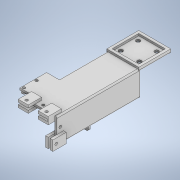
# Autodesk Inventor part: carriageEndL
Saved by Autodesk Inventor 2020 (Build 240168000, 168)
## iProperties
Created: 2020-01-10
Part Number: carriageEndL
Material: Generic
Document SubType Name: Modeling
Designer: PAB
Density: 1 g/cm^3
Appearance: Default
Author: PAB
Autodesk Inventor part; units mm, degrees
ref_plane "YZ Plane" through (0, 0, 0) normal (1, 0, 0) x (0, 1, 0)
ref_plane "XZ Plane" through (0, 0, 0) normal (0, 1, 0) x (-1, 0, 0)
ref_plane "XY Plane" through (0, 0, 0) normal (0, 0, 1) x (1, 0, 0)
sketch "Sketch1" plane through (0, 0, 0) normal (0, 1, 0) x (-1, 0, 0)
  line L0 (24, 138) -> (-24, 138)
  line L1 (-24, 138) -> (-24, -138)
  line L2 (-24, -138) -> (24, -138)
  line L3 (24, -138) -> (24, 138)
  point P0 (0, 0)
  dimension "d0" = 48
  dimension "d1" = 276
  constraints: 8 end point, 2 parallel, 1 horizontal, 1 perpendicular
  measures "d0" distance of L2.end L1.end
  measures "d1" distance of L1.end L0.end
extrude "Extrusion1" add sketch "Sketch1" along normal blind 3
sketch "Sketch2" plane through (0, 3, 0) normal (0, 1, 0) x (1, 0, 0)
  line L0 (-24, 138) -> (-24, -138) projected
  line L1 (-24, -138) -> (-20, -138)
  line L2 (-20, -138) -> (-20, -90)
  line L3 (-20, -90) -> (-24, -90)
  line L4 (-24, -90) -> (-24, -138)
  line L5 (24, -138) -> (24, 138) projected
  line L6 (-20, -90) -> (24, -90)
  line L7 (24, -90) -> (24, -94)
  line L8 (24, -94) -> (-20, -94)
  line L9 (-20, -94) -> (-20, -90)
  line L10 (-24, -138) -> (24, -138) projected
  line L11 (24, -94) -> (20, -94)
  line L12 (20, -94) -> (20, -138)
  line L13 (20, -138) -> (24, -138)
  line L14 (24, -138) -> (24, -94)
  line L15 (20, -138) -> (-20, -138)
  line L16 (-20, -138) -> (-20, -134)
  line L17 (-20, -134) -> (20, -134)
  line L18 (20, -134) -> (20, -138)
  point P0 (0, 0)
  point P1 (20, -134)
  dimension "d4" = 4
  dimension "d5" = 48
  dimension "d6" = 4
  dimension "d7" = 4
  dimension "d8" = 4
  constraints: 32 end point, 8 parallel, 4 horizontal, 4 perpendicular, 3 point on line
  measures "d4" distance of L3.end L2.end
  measures "d5" distance of L2.end L1.end
  measures "d6" distance of L6.end L7.end
  measures "d7" distance of L13.end L12.end
  measures "d8" distance of L15.end L16.end
extrude "Extrusion2" add sketch "Sketch2" along normal blind 3 contours L3 L2 L1 L0 | L6 L5 L8 L2 | L2 L17 L12 L10 | L12 L8 L5 L10
mirror "Mirror1" about plane through (0, 0, 0) normal (0, 0, 1) of "Extrusion2"
sketch "Sketch3" plane through (0, 0, 0) normal (0, -1, 0) x (1, 0, 0)
  line L0 (24, -90) -> (-24, -90) projected
  line L1 (24, 138) -> (24, -138) projected
  line L2 (-24, -90) -> (24, -90)
  line L3 (24, -90) -> (24, -93)
  line L4 (24, -93) -> (-24, -93)
  line L5 (-24, -93) -> (-24, -90)
  line L6 (-24, 90) -> (24, 90) projected
  line L7 (24, 90) -> (21, 90)
  line L8 (21, 90) -> (21, -90)
  line L9 (21, -90) -> (24, -90)
  line L10 (24, -90) -> (24, 90)
  line L11 (-24, 90) -> (24, 90)
  line L12 (24, 90) -> (24, 93)
  line L13 (24, 93) -> (-24, 93)
  line L14 (-24, 93) -> (-24, 90)
  point P0 (0, 0)
  dimension "d11" = 3
  dimension "d12" = 3
  dimension "d13" = 3
  constraints: 24 end point, 6 parallel, 3 horizontal, 3 perpendicular, 3 point on line
  measures "d11" distance of L2.end L3.end
  measures "d12" distance of L9.end L8.end
  measures "d13" distance of L12.end L11.end
extrude "Extrusion3" add sketch "Sketch3" along normal blind 35
sketch "Sketch4" plane through (-24, 0, -90) normal (0, 0, 1) x (1, 0, 0)
  line L0 (0, -35) -> (45, -35) projected
  line L1 (45, 0) -> (45, -35) projected
  line L2 (0, -35) -> (45, -35)
  line L3 (45, -35) -> (45, -31)
  line L4 (45, -31) -> (0, -31)
  line L5 (0, -31) -> (0, -35)
  point P0 (24, 0)
  dimension "d16" = 4
  constraints: 8 end point, 2 parallel, 1 horizontal, 1 perpendicular, 1 point on line
  measures "d16" distance of L3.end L2.end
extrude "Extrusion4" add sketch "Sketch4" along normal blind 8
sketch "Sketch5" plane through (-24, -31, -90) normal (0, 1, 0) x (1, 0, 0)
  line L0 (0, -8) -> (45, -8) projected
  line L1 (45, 0) -> (45, -8) projected
  line L2 (0, -8) -> (45, -8)
  line L3 (45, -8) -> (45, -4)
  line L4 (45, -4) -> (0, -4)
  line L5 (0, -4) -> (0, -8)
  point P0 (24, -90)
  dimension "d19" = 4
  constraints: 8 end point, 2 parallel, 1 horizontal, 1 midpoint, 1 perpendicular
  measures "d19" distance of L3.end L2.end
extrude "Extrusion5" add sketch "Sketch5" along normal blind 4
sketch "Sketch6" plane through (0, 0, 0) normal (0, -1, 0) x (1, 0, 0)
  line L0 (21, -86) -> (-24, -86) projected
  line L1 (-24, -82) -> (21, -82)
  line L2 (21, -82) -> (21, -86)
  line L3 (21, -86) -> (-24, -86)
  line L4 (-24, -86) -> (-24, -82)
  point P0 (0, 0)
  dimension "d22" = 4
  constraints: 8 end point, 2 parallel, 1 horizontal, 1 perpendicular
  measures "d22" distance of L1.end L0.start
extrude "Extrusion6" add sketch "Sketch6" along normal blind 4
mirror "Mirror2" about plane through (0, 0, 0) normal (0, 0, 1) of "Extrusion6", "Extrusion5", "Extrusion4"
sketch "Sketch7" plane through (0, 0, 0) normal (0, -1, 0) x (1, 0, 0)
  circle A0 centre (-14, -127) radius 3
  circle A1 centre (14, -127) radius 3
  circle A2 centre (14, -101) radius 3
  circle A3 centre (-14, -101) radius 3
  line L0 (-20, -94) -> (20, -94) projected
  line L1 (20, -94) -> (20, -134) projected
  line L2 (-20, -134) -> (-20, -94) projected
  point P0 (0, 0)
  dimension "d25" = 6
  dimension "d26" = 6
  dimension "d27" = 6
  dimension "d28" = 6
  dimension "d135" = 28
  dimension "d136" = 26
  dimension "d137" = 28
  dimension "d138" = 26
  dimension "d139" = 7
  dimension "d140" = 7
  dimension "d141" = 6
  dimension "d142" = 6
  constraints: 4 centre point
  measures "d25" diameter of A0
  measures "d26" diameter of A1
  measures "d27" diameter of A2
  measures "d28" diameter of A3
  measures "d135" distance of A2.centre A3.centre
  measures "d136" distance of A1.centre A2.centre
  measures "d137" distance of A1.centre A0.centre
  measures "d138" distance of A3.centre A0.centre
  measures "d139" distance from line of L0 A3.centre
  measures "d140" distance from line of L0 A2.centre
  measures "d141" distance from line of L1 A2.centre
  measures "d142" distance from line of L2 A0.centre
extrude "Extrusion7" cut sketch "Sketch7" against normal blind 4
mirror "Mirror3" about plane through (0, 0, 0) normal (0, 0, 1) of "Extrusion7"
sketch "Sketch8" plane through (0, 0, 0) normal (0, -1, 0) x (1, 0, 0)
  line L0 (21, 82) -> (21, -82) projected
  line L1 (-24, -82) -> (-24, 82) projected
  line L2 (21, -20) -> (-24, -20)
  line L3 (-24, -20) -> (-24, -17)
  line L4 (-24, -17) -> (21, -17)
  line L5 (21, -17) -> (21, -20)
  point P0 (0, 0)
  dimension "d31" = 3
  constraints: 8 end point, 2 parallel, 2 point on line, 1 horizontal, 1 perpendicular
  measures "d31" distance of L2.end L3.end
extrude "Extrusion8" add sketch "Sketch8" along normal blind 42.3
sketch "Sketch9" plane through (21, 0, -20) normal (0, 0, -1) x (-1, 0, 0)
  circle A0 centre (39.35, -5.65) radius 4
  circle A1 centre (39.35, -36.65) radius 4
  circle A2 centre (8.35, -5.65) radius 4
  circle A3 centre (8.35, -36.65) radius 4
  point P0 (21, 0)
  dimension "d34" = 8
  dimension "d35" = 8
  dimension "d36" = 8
  dimension "d37" = 8
  constraints: 4 centre point
  measures "d34" diameter of A0
  measures "d35" diameter of A1
  measures "d36" diameter of A2
  measures "d37" diameter of A3
extrude "Extrusion9" add sketch "Sketch9" along normal blind 3
sketch "Sketch10" plane through (-18.35, -36.65, -23) normal (0, 0, -1) x (-1, 0, 0)
  circle A0 centre (0, 0) radius 3
  circle A1 centre (0, 31) radius 4 projected
  circle A2 centre (0, 31) radius 3
  circle A3 centre (-31, 0) radius 4 projected
  circle A4 centre (-31, 0) radius 3
  circle A5 centre (-31, 31) radius 4 projected
  circle A6 centre (-31, 31) radius 3
  point P0 (-18.35, 36.65)
  dimension "d40" = 6
  dimension "d41" = 6
  dimension "d42" = 6
  dimension "d43" = 6
  constraints: 4 centre point, 3 coincident
  measures "d40" diameter of A0
  measures "d41" diameter of A2
  measures "d42" diameter of A4
  measures "d43" diameter of A6
extrude "Extrusion10" cut sketch "Sketch10" against normal blind 2 contours A0 | A2 | A4 | A6
sketch "Sketch11" plane through (21, 0, -20) normal (0, 0, -1) x (-1, 0, 0)
  circle A0 centre (23.85, -21.15) radius 12.5
  circle A1 centre (39.35, -36.65) radius 3 projected
  circle A2 centre (39.35, -36.65) radius 2
  circle A3 centre (8.35, -36.65) radius 3 projected
  circle A4 centre (8.35, -36.65) radius 2
  circle A5 centre (8.35, -5.65) radius 4 projected
  circle A6 centre (8.35, -5.65) radius 2
  circle A7 centre (39.35, -5.65) radius 4 projected
  circle A8 centre (39.35, -5.65) radius 2
  point P0 (21, 0)
  dimension "d46" = 25
  dimension "d47" = 4
  dimension "d48" = 4
  dimension "d49" = 4
  dimension "d50" = 4
  constraints: 5 centre point, 4 coincident
  measures "d46" diameter of A0
  measures "d47" diameter of A2
  measures "d48" diameter of A4
  measures "d49" diameter of A6
  measures "d50" diameter of A8
extrude "Extrusion11" cut sketch "Sketch11" along normal mid plane 10 contours A0 | A2 | A4 | A6 | A8
sketch "Sketch20" plane through (0, 0, 0) normal (0, -1, 0) x (1, 0, 0)
  line L0 (-24, -90) -> (-24, 90) projected
  line L1 (-24, 138) -> (24, 138) projected
  line L2 (-24, 33) -> (24, 33)
  line L3 (24, 33) -> (24, 138)
  line L4 (24, 138) -> (-24, 138)
  line L5 (-24, 138) -> (-24, 33)
  point P0 (0, 0)
  constraints: 8 end point, 2 parallel, 1 horizontal, 1 perpendicular, 1 point on line
extrude "Extrusion20" cut sketch "Sketch20" along normal mid plane 100
sketch "Sketch21" plane through (0, 0, 0) normal (0, -1, 0) x (1, 0, 0)
  line L0 (-24, 23) -> (-9, 23)
  line L1 (-9, 23) -> (-9, 43)
  line L2 (-9, 43) -> (-24, 43)
  line L3 (-24, 43) -> (-24, 23)
  line L4 (6, 23) -> (21, 23)
  line L5 (21, 23) -> (21, 43)
  line L6 (21, 43) -> (6, 43)
  line L7 (6, 43) -> (6, 23)
  point P0 (0, 0)
  dimension "d86" = 15
  dimension "d87" = 20
  dimension "d88" = 15
  dimension "d89" = 20
  constraints: 16 end point, 4 parallel, 2 horizontal, 2 perpendicular
  measures "d86" distance of L2.end L1.end
  measures "d87" distance of L1.end L0.end
  measures "d88" distance of L6.end L5.end
  measures "d89" distance of L5.end L4.end
extrude "Extrusion21" add sketch "Sketch21" along normal blind 4 and the other way blind 7
sketch "Sketch24" plane through (0, -4, 0) normal (0, -1, 0) x (1, 0, 0)
  circle A0 centre (-16.5, 38) radius 2
  circle A1 centre (13.5, 38) radius 2
  circle A2 centre (-1.5, 28) radius 2
  point P0 (0, 0)
  dimension "d102" = 4
  dimension "d103" = 4
  dimension "d104" = 4
  constraints: 3 centre point
  measures "d102" diameter of A0
  measures "d103" diameter of A1
  measures "d104" diameter of A2
extrude "Extrusion24" cut sketch "Sketch24" against normal blind 15
sketch "Sketch25" plane through (21, -35, -17) normal (-1, 0, 0) x (0, 0, 1)
  line L0 (-76, 0) -> (50, 0) projected
  line L1 (40, 0) -> (60, 0)
  line L2 (60, 0) -> (60, 15)
  line L3 (60, 15) -> (40, 15)
  line L4 (40, 15) -> (40, 0)
  point P0 (17, 35)
  point P1 (50, 0)
  dimension "d107" = 20
  dimension "d108" = 15
  constraints: 8 end point, 2 parallel, 1 horizontal, 1 perpendicular, 1 point on line
  measures "d107" distance of L3.end L2.end
  measures "d108" distance of L2.end L1.end
extrude "Extrusion25" add sketch "Sketch25" along normal blind 4 and the other way blind 7
sketch "Sketch26" plane through (6, -4, 43) normal (0, 0, 1) x (1, 0, 0)
  line L0 (18, 4) -> (-30, 4) projected
  line L1 (14, 7) -> (14, 10) projected
  line L2 (-30, 4) -> (14, 4)
  line L3 (14, 4) -> (14, 7)
  line L4 (14, 7) -> (-30, 7)
  line L5 (-30, 7) -> (-30, 4)
  line L6 (15, -31) -> (15, -38.3) projected
  line L7 (22, -16) -> (18, -16) projected
  line L8 (15, -31) -> (18, -31)
  line L9 (18, -31) -> (18, -16)
  line L10 (18, -16) -> (15, -16)
  line L11 (15, -16) -> (15, -31)
  point P0 (-6, 4)
  constraints: 16 end point, 4 parallel, 2 horizontal, 2 perpendicular
extrude "Extrusion26" cut sketch "Sketch26" against normal blind 10
sketch "Sketch27" plane through (21, -35, -17) normal (-1, 0, 0) x (0, 0, 1)
  circle A0 centre (55, 7.5) radius 2
  circle A1 centre (45, 22.5) radius 2
  point P0 (17, 35)
  dimension "d117" = 4
  dimension "d118" = 4
  constraints: 2 centre point
  measures "d117" diameter of A0
  measures "d118" diameter of A1
extrude "Extrusion27" cut sketch "Sketch27" along normal mid plane 20
sketch "Sketch28" plane through (-24, 0, -138) normal (-1, 0, 0) x (0, 0, 1)
  line L0 (161, 3) -> (171, 3) projected
  line L1 (121, 0) -> (161, 0) projected
  line L2 (161, 3) -> (121, 3)
  line L3 (121, 3) -> (121, 0)
  line L4 (121, 0) -> (161, 0)
  line L5 (161, 0) -> (161, 3)
  point P0 (138, 0)
  dimension "d123" = 40
  constraints: 8 end point, 2 parallel, 1 horizontal, 1 perpendicular
  measures "d123" distance of L4.end L1.start
extrude "Extrusion28" add sketch "Sketch28" along normal blind 17.5
sketch "Sketch29" plane through (0, 0, 0) normal (0, -1, 0) x (1, 0, 0)
  circle A0 centre (-38.5, 20) radius 3
  circle A1 centre (-38.5, 1) radius 3
  point P0 (0, 0)
  dimension "d126" = 6
  dimension "d127" = 6
  constraints: 2 centre point
  measures "d126" diameter of A0
  measures "d127" diameter of A1
extrude "Extrusion29" add sketch "Sketch29" along normal blind 3
sketch "Sketch30" plane through (-38.5, -3, 20) normal (0, -1, 0) x (1, 0, 0)
  circle A0 centre (0, 0) radius 2
  circle A1 centre (0, -19) radius 3 projected
  circle A2 centre (0, -19) radius 2
  point P0 (38.5, -20)
  point P1 (-3, -19)
  dimension "d130" = 4
  dimension "d131" = 4
  constraints: 2 centre point, 1 coincident, 1 horizontal alignment
  measures "d130" diameter of A0
  measures "d131" diameter of A2
extrude "Extrusion30" cut sketch "Sketch30" against normal blind 10 contours A0 | A2
fillet "Fillet3" radius 2 10 edges at (24, -35, -35) (0, -35, -93) (21, -42.3, -18.5) (-24, -42.3, -18.5) (24, 0, -115.5) (0, 0, -138) (-24, 0, -115.5) (24, 3, -28.5) (-24, 3, -53.5) (24, -17.5, -93)
body "Solid1"
